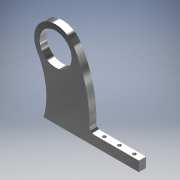
# Autodesk Inventor part: Idle Shooter holder
Saved by Autodesk Inventor 2019.4 (Build 234330000, 330)
## iProperties
Created: 2020-01-11
Part Number: Idle Shooter holder
Material: Aluminum 6061
Document SubType Name: Modeling
Designer: admin
Density: 2.7 g/cm^3
Appearance: Aluminum - Flat
Author: admin
Autodesk Inventor part; units mm, degrees
ref_plane "YZ Plane" through (0, 0, 0) normal (1, 0, 0) x (0, 1, 0)
ref_plane "XZ Plane" through (0, 0, 0) normal (0, 1, 0) x (-1, 0, 0)
ref_plane "XY Plane" through (0, 0, 0) normal (0, 0, 1) x (1, 0, 0)
sketch "Sketch1" plane through (0, 0, 0) normal (0, 0, 1) x (1, 0, 0)
  circle A0 centre (0, 0) radius 16
  arc A1 (-18.6289, -10.7337) -> (18.6289, 10.7337) centre (0, 0) ccw construction
  arc A2 (-12, -65) -> (-18.6289, -10.7337) centre (-79.2813, -45.6808) ccw
  arc A3 (33.3338, -55) -> (18.6289, 10.7337) centre (-79.2813, -45.6808) ccw
  line L0 (33.3338, -55) -> (83.3338, -55)
  line L1 (83.3338, -55) -> (83.3338, -65)
  line L2 (83.3338, -65) -> (-12, -65)
  arc A4 (18.6289, 10.7337) -> (-18.6289, -10.7337) centre (0, 0) ccw
  dimension "d0" = 32
  dimension "d1" = 43
  dimension "d2" = 10
  dimension "d3" = 65
  dimension "d4" = 70
  dimension "d5" = 50
  dimension "d6" = 12
  constraints: 8 point on circle, 6 end point, 5 centre point, 3 coincident, 2 perpendicular, 2 tangent, 1 horizontal
  measures "d0" diameter of A0
  measures "d1" diameter of A1
  measures "d2" distance of L0.end L1.end
  measures "d3" distance from line of point (0, 0) L2
  measures "d4" radius of A2
  measures "d5" distance of L0.start L0.end
  measures "d6" horizontal distance of L2.end point (0, 0)
extrude "Extrusion1" add sketch "Sketch1" along normal blind 7
fillet "Fillet1" radius 5 1 edges at (33.3338, -55, 3.5)
sketch "Sketch2" plane through (83.3338, -55, 7) normal (0, 1, 0) x (1, 0, 0)
  circle A0 centre (-38, 3.5) radius 1.75
  circle A1 centre (-23, 3.5) radius 1.75
  circle A2 centre (-8, 3.5) radius 1.75
  line L0 (-8, 3.5) -> (-38, 3.5) construction
  line L1 (0, 7) -> (0, 0) projected
  line L2 (0, 7) -> (-44.6941, 7) projected
  point P0 (-83.3338, 7)
  dimension "d10" = 3.5
  dimension "d11" = 3.5
  dimension "d12" = 3.5
  dimension "d13" = 30
  dimension "d14" = 8
  dimension "d15" = 3.5
  constraints: 3 centre point, 2 end point, 1 coincident, 1 horizontal, 1 midpoint
  measures "d10" diameter of A0
  measures "d11" diameter of A1
  measures "d12" diameter of A2
  measures "d13" distance of L0.start L0.end
  measures "d14" distance from line of L1 L0.start
  measures "d15" distance between parallel lines of L2 L0
extrude "Extrusion2" cut sketch "Sketch2" against normal through all
equation "\"d11\" = d10"
equation "\"d12\" = d10"
body "Solid1"
